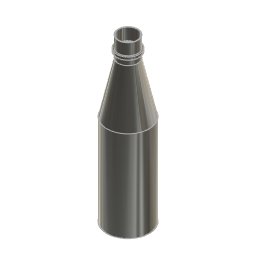
Q2 Bottle (Autodesk Fusion 360 archive; units mm, degrees)
design "Bottle"
Autodesk Fusion 360 part; units mm, degrees
sketch "Sketch1" plane through (0, 0, 0) normal (1, 0, 0) x (0, 1, 0)
  line L0 (0, 0) -> (3.75, 0)
  line L1 (0, 0) -> (-3.75, 0)
  line L2 (3.75, 0) -> (3.75, 16)
  line L3 (-3.75, 0) -> (-3.75, 16)
  line L4 (-1.75, 25) -> (-1.75, 26)
  line L5 (1.75, 25) -> (1.75, 26)
  line L6 (-1.75, 25) -> (-3.75, 16)
  line L7 (1.75, 25) -> (3.75, 16)
  line L8 (1.75, 26) -> (2, 26)
  line L9 (2, 26) -> (2, 26.5)
  line L10 (2, 26.5) -> (1.75, 26.5)
  line L11 (1.75, 26.5) -> (1.75, 28.5)
  line L12 (1.75, 28.5) -> (-1.75, 28.5)
  line L13 (-1.75, 28.5) -> (-1.75, 26.5)
  line L14 (-1.75, 26.5) -> (-2, 26.5)
  line L15 (-2, 26.5) -> (-2, 26)
  line L16 (-2, 26) -> (-1.75, 26)
  line L17 (0, 0) -> (0, 28.5)
  dimension "d1" = 3.75
  dimension "d2" = 3.75
  dimension "d3" = 16
  dimension "d4" = 16
  dimension "d7" = 3.5
  dimension "d10" = 0.25
  dimension "d11" = 0.5
  dimension "d12" = 2
  constraint coincident L0.start L1.start
  constraint horizontal L0
  constraint parallel L0 L1
  constraint perpendicular L0 L2
  constraint perpendicular L1 L3
  constraint perpendicular L5 L8
  constraint perpendicular L8 L9
  constraint perpendicular L9 L10
  constraint perpendicular L10 L11
  constraint perpendicular L11 L12
  constraint horizontal L12
  constraint perpendicular L12 L13
  constraint perpendicular L13 L14
  constraint perpendicular L14 L15
  constraint perpendicular L4 L16
  constraint midpoint L12 L17.end
  measures "d1" distance of L0.start L0.end
  measures "d2" distance of L0.start L1.end
  measures "d3" distance of L0.end L2.end
  measures "d4" distance of L1.end L3.end
  measures "d7" distance of L11.end L12.end
  measures "d10" distance of L9.end L10.end
  measures "d11" distance of L8.end L9.end
  measures "d12" distance of L10.end L11.end
revolve "Revolve1" add sketch "Sketch1" angle 360 about axis through (0, 0, 0) along (0, 0, 1) contours L0 L2 L5 L7 L8 L9 L10 L11 L12 L17
shell "Shell1" thickness 0.1 removed faces 1 at (-0.8743, -0.5048, 28.5)
equation "d1 = ( 7.5 / 2 ) * 1 mm"

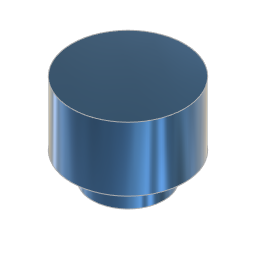
design "Cap"
Autodesk Fusion 360 part; units mm, degrees
sketch "Sketch1" plane through (0, 0, 0) normal (0, 1, 0) x (1, 0, 0)
  line L0 (1.75, 0) -> (2.2, 0)
  line L1 (-1.75, 0) -> (-2.2, 0)
  line L2 (2.2, 0) -> (2.2, -2.5)
  line L3 (-2.2, 0) -> (-2.2, -2.5)
  line L4 (-2.2, -2.5) -> (2.2, -2.5)
  line L5 (1.75, 0) -> (1.75, -2)
  line L6 (-1.75, 0) -> (-1.75, -2)
  line L7 (-1.75, -2) -> (-1.6, -2)
  line L8 (-1.6, -2) -> (-1.6, 0.3)
  line L9 (-1.6, 0.3) -> (-1.4, 0.3)
  line L10 (-1.4, 0.3) -> (-1.4, 1)
  line L11 (1.75, -2) -> (1.6, -2)
  line L12 (1.6, -2) -> (1.6, 0.3)
  line L13 (1.6, 0.3) -> (1.4, 0.3)
  line L14 (1.4, 0.3) -> (1.4, 1)
  line L15 (1.4, 1) -> (-1.4, 1)
  line L16 (0, -2.5) -> (0, 1)
  dimension "d1" = 1.75
  dimension "d2" = 1.75
  dimension "d3" = 0.45
  dimension "d4" = 2.5
  dimension "d5" = 2.5
  constraint perpendicular L0 L2
  constraint perpendicular L1 L3
  constraint perpendicular L2 L4
  constraint perpendicular L0 L5
  constraint perpendicular L1 L6
  constraint perpendicular L6 L7
  constraint perpendicular L7 L8
  constraint perpendicular L8 L9
  constraint perpendicular L9 L10
  constraint perpendicular L5 L11
  constraint perpendicular L11 L12
  constraint perpendicular L12 L13
  constraint perpendicular L13 L14
  constraint perpendicular L10 L15
  constraint collinear L9 L13
  constraint midpoint L4 L16.start
  constraint midpoint L15 L16.end
  measures "d1" distance of origin L0.start
  measures "d2" distance of origin L1.start
  measures "d3" distance of L0.start L0.end
  measures "d4" distance of L0.end L2.end
  measures "d5" distance of L1.end L3.end
revolve "Revolve1" add sketch "Sketch1" angle 360 about axis through (0, 0, 2.5) along (0, 0, -1) contours L0 L2 L4 L5 L11 L12 L13 L14 L15 L16
equation "d1 = ( 3.5 / 2 ) * 1 mm"
equation "d2 = ( 3.5 / 2 ) * 1 mm"
